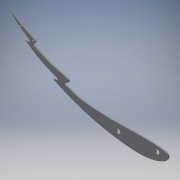
# Autodesk Inventor part: newbracket2
Saved by Autodesk Inventor 2018 (Build 220112000, 112)
## iProperties
Created: 2018-06-13
Part Number: newbracket2
Material: 一般
Document SubType Name: Modeling
Designer: ku_sk
Density: 1 g/cm^3
Appearance: 既定
Author: ku_sk
Autodesk Inventor part; units mm, degrees
ref_plane "YZ Plane" through (0, 0, 0) normal (1, 0, 0) x (0, 1, 0)
ref_plane "XZ Plane" through (0, 0, 0) normal (0, 1, 0) x (-1, 0, 0)
ref_plane "XY Plane" through (0, 0, 0) normal (0, 0, 1) x (1, 0, 0)
sketch "スケッチ1" plane through (0, 0, 0) normal (0, 1, 0) x (-1, 0, 0)
  arc A0 (395.0712, 101.8969) -> (435.2675, 137.2475) centre (306.3013, 243.3635) ccw
  arc A1 (365.0957, 97.3477) -> (365.7216, 93.5054) centre (366.6087, 95.622) ccw
  arc A2 (369.5386, 100.605) -> (365.0957, 97.3477) centre (385.9519, 73.5593) ccw
  arc A3 (385.8674, 109.4763) -> (369.5386, 100.605) centre (470.4646, -65.7001) ccw
  arc A4 (385.8674, 109.4763) -> (396.1841, 114.479) centre (-1159.575, 3309.6389) ccw
  arc A5 (396.1841, 114.479) -> (414.939, 124.7316) centre (296.9263, 318.331) ccw
  arc A6 (414.939, 124.7316) -> (434.3408, 138.1953) centre (311.0977, 295.0828) ccw
  arc A7 (435.2675, 137.2475) -> (434.3408, 138.1953) centre (434.7527, 137.6711) ccw
  arc A8 (319.6761, 45.1314) -> (390.0033, 84.5371) centre (233.4832, 281.4189) ccw
  arc A9 (273.0796, 42.1444) -> (277.153, 40.2312) centre (280.7432, 53.1684) ccw
  arc A10 (273.4497, 49.6709) -> (273.0796, 42.1444) centre (275.6154, 45.792) ccw
  arc A11 (281.147, 53.127) -> (273.4497, 49.6709) centre (297.0704, 7.3635) ccw
  arc A12 (307.9726, 61.0464) -> (281.147, 53.127) centre (377.3682, -223.4121) ccw
  arc A13 (307.9726, 61.0464) -> (324.6713, 65.1488) centre (-955.196, 5238.8807) ccw
  circle A14 centre (20.1088, -0.8575) radius 6
  circle A15 centre (130.7072, -5.574) radius 6
  arc A16 (390.0033, 84.5371) -> (388.4453, 88.078) centre (388.7587, 86.1027) ccw
  line L0 (388.4453, 88.078) -> (384.6663, 87.4784)
  arc A17 (382.4737, 92.8975) -> (384.6663, 87.4784) centre (384.1962, 90.4413) ccw
  arc A18 (281.147, 53.127) -> (273.4497, 49.6709) centre (297.0704, 7.3635) ccw
  line L1 (277.153, 40.2312) -> (280.996, 39.1647)
  arc A19 (281.136, 33.4257) -> (280.996, 39.1647) centre (280.1938, 36.274) ccw
  line L2 (281.136, 33.4257) -> (251.9878, 23.784)
  arc A20 (232.2409, 19.4065) -> (251.9878, 23.784) centre (220.5829, 118.7246) ccw
  arc A21 (202.438, 16.5387) -> (232.2409, 19.4065) centre (148.7903, 730.3461) ccw
  arc A22 (125.7464, 14.4013) -> (202.438, 16.5387) centre (141.4444, 828.0876) ccw
  arc A23 (84.4867, 15.2639) -> (125.7464, 14.4013) centre (372.4747, 12803.2702) ccw
  arc A24 (84.4867, 15.2639) -> (17.3799, 13.5681) centre (68.6653, -687.2803) ccw
  arc A25 (17.3799, 13.5681) -> (-2.611, 10.3374) centre (25.867, -102.4131) ccw
  arc A26 (-2.611, 10.3374) -> (-8.1443, -6.881) centre (0, 0) ccw
  arc A27 (-8.1443, -6.881) -> (0.1105, -13.8465) centre (16.4695, 13.9147) ccw
  arc A28 (0.1105, -13.8465) -> (28.2747, -25.3165) centre (53.2618, 76.3513) ccw
  arc A29 (28.2747, -25.3165) -> (76.0298, -30.4027) centre (70.8911, 148.0818) ccw
  arc A30 (76.0298, -30.4027) -> (101.7324, -28.9004) centre (63.5115, 404.3974) ccw
  arc A31 (101.7324, -28.9004) -> (312.4116, 29.4193) centre (48.6916, 572.4065) ccw
  arc A32 (312.4116, 29.4193) -> (311.5978, 33.2175) centre (311.5379, 31.2183) ccw
  line L3 (311.5978, 33.2175) -> (304.4845, 33.4306)
  arc A33 (303.5463, 39.2476) -> (304.4845, 33.4306) centre (304.5744, 36.4292) ccw
  line L4 (303.5463, 39.2476) -> (319.6761, 45.1314)
  line L5 (365.7216, 93.5054) -> (369.4507, 91.9425)
  arc A34 (369.4958, 84.5835) -> (369.4507, 91.9425) centre (367.9046, 88.2534) ccw
  line L6 (369.4958, 84.5835) -> (324.6713, 65.1488)
  line L7 (395.0712, 101.8969) -> (382.4737, 92.8975)
  point P0 (0, 0)
  dimension "d1" = 4
  constraints: 66 point on circle, 35 centre point, 16 end point, 3 tangent
  measures "d1" radius of A34
extrude "押し出し2" add sketch "スケッチ1" along normal mid plane 4
sketch "スケッチ2" plane through (0, -2, 0) normal (0, -1, 0) x (1, 0, 0)
  circle A0 centre (-372.2064, 97.2423) radius 3.25
  circle A1 centre (-405.9401, 114.7361) radius 3.25
  line L0 (-405.9401, 114.7361) -> (-372.2064, 97.2423)
  point P0 (0, 0)
  dimension "d6" = 6.5
  dimension "d7" = 6.5
  dimension "d8" = 38
  constraints: 2 centre point, 2 end point
  measures "d6" diameter of A1
  measures "d7" diameter of A0
  measures "d8" distance of L0.start L0.end
extrude "押し出し3" cut sketch "スケッチ2" against normal blind 10
